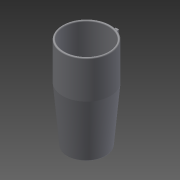
# Autodesk Inventor part: EDF Cone
Saved by Autodesk Inventor 2014 SP1 (Build 180222100, 222)
## iProperties
Created: 2018-05-08
Part Number: EDF Cone
Material: Generic
Document SubType Name: Modeling
Designer: Dadang
Density: 1 g/cm^3
Appearance: Default
Author: Dadang
Autodesk Inventor part; units mm, degrees
ref_plane "YZ Plane" through (0, 0, 0) normal (1, 0, 0) x (0, 1, 0)
sketch "Sketch1" plane through (0, 0, 0) normal (0, 0, 1) x (1, 0, 0)
  circle A0 centre (0, 0) radius 35
  dimension "d0" = 70
  constraints: 1 centre point, 1 coincident
  measures "d0" diameter of A0
extrude "Extrusion1" add sketch "Sketch1" along normal blind 55
ref_plane "Work Plane1" through (0, 0, -80) normal (0, 0, 1) x (1, 0, 0)
sketch "Sketch2" plane through (0, 0, -80) normal (0, 0, 1) x (1, 0, 0)
  circle A0 centre (0, 0) radius 28
  dimension "d4" = 56
  constraints: 1 centre point, 1 coincident
  measures "d4" diameter of A0
loft "Loft1" add profiles "Sketch2" section 1 edges at (-35, 0, 0)
shell "Shell1" thickness 3 removed faces 2 at (1.125, 3.113, -80) at (-1.9985, 11.019, 55)
ref_plane "Work Plane3" through (0, 35, 0) normal (0, 1, 0) x (-1, 0, 0)
sketch "Sketch3" plane through (0, 35, 0) normal (0, 1, 0) x (-1, 0, 0)
  line L0 (35, 55) -> (-35, 55) projected
  line L1 (2.5, 10) -> (2.5, 45)
  line L2 (2.5, 45) -> (-2.5, 45)
  line L3 (2.5, 10) -> (-2.5, 10)
  line L4 (-2.5, 10) -> (-2.5, 45)
  point P0 (0, 0)
  dimension "d15" = 5
  dimension "d18" = 5
  constraints: 8 end point, 1 perpendicular
  measures "d15" distance of L1.end L2.end
  measures "d18" distance of L1.start L3.end
extrude "Extrusion2" add sketch "Sketch3" along normal blind 10
fillet "Fillet1" radius 1.5 4 edges at (-35, 0, 55) (-32, 0, 55) (-28, 0, -80) (-24.9885, 0, -80)
body "Solid1"
